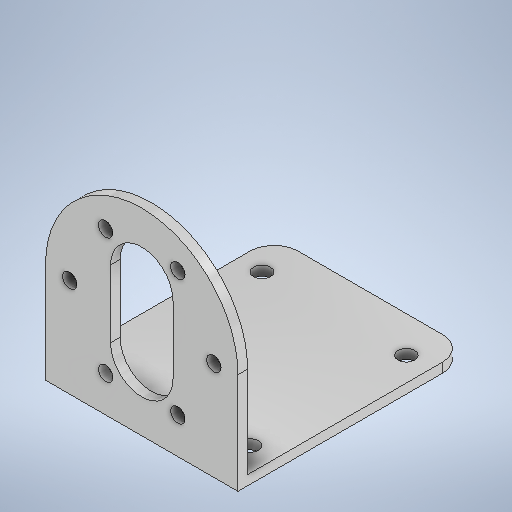
# Autodesk Inventor part: 520 DC Gear Motor Bracket
Saved by Autodesk Inventor 2025.2 (Build 292293000, 293)
## iProperties
Created: 2025-01-16
Part Number: 520 DC Gear Motor Bracket
Material: Generic
Document SubType Name: Modeling
Designer: Matt Tidd
Density: 1 g/cm^3
Appearance: Default
Author: Matt Tidd
Autodesk Inventor part; units mm, degrees
ref_plane "YZ Plane" through (0, 0, 0) normal (1, 0, 0) x (0, 1, 0)
ref_plane "XZ Plane" through (0, 0, 0) normal (0, 1, 0) x (-1, 0, 0)
ref_plane "XY Plane" through (0, 0, 0) normal (0, 0, 1) x (1, 0, 0)
sketch "Sketch1" plane through (0, 0, 0) normal (1, 0, 0) x (0, 1, 0)
  line L0 (0, 0) -> (2, 0)
  line L1 (2, 0) -> (2, -47.5)
  line L2 (2, -47.5) -> (0, -47.5)
  line L3 (0, -47.5) -> (0, 0)
  line L4 (0, 0) -> (41, 0)
  line L5 (41, 0) -> (41, -2)
  line L6 (41, -2) -> (0, -2)
  line L7 (0, -2) -> (0, 0)
  point P0 (2, -2)
  dimension "d0" = 2
  dimension "d1" = 47.5
  dimension "d2" = 41
  dimension "d3" = 2
  constraints: 16 end point, 4 parallel, 2 horizontal, 2 perpendicular
  measures "d0" distance of L1.end L2.end
  measures "d1" distance of L0.end L1.end
  measures "d2" distance of L5.end L6.end
  measures "d3" distance of L4.end L5.end
extrude "Extrusion1" add sketch "Sketch1" along normal blind 40
sketch "Sketch2" plane through (0, 0, 0) normal (0, 0, 1) x (1, 0, 0)
  line L0 (20, 27.5) -> (20, 13.5) construction
  line L1 (13.5, 27.5) -> (13.5, 13.5)
  line L2 (26.5, 13.5) -> (26.5, 27.5)
  arc A0 (26.5, 27.5) -> (13.5, 27.5) centre (20, 27.5) ccw
  arc A1 (13.5, 13.5) -> (26.5, 13.5) centre (20, 13.5) ccw
  circle A2 centre (35, 20.5) radius 1.5
  circle A3 centre (27.5, 33.4904) radius 1.5
  circle A4 centre (12.5, 33.4904) radius 1.5
  circle A5 centre (5, 20.5) radius 1.5
  circle A6 centre (12.5, 7.5096) radius 1.5
  circle A7 centre (27.5, 7.5096) radius 1.5
  point P0 (0, 0)
  point P1 (20, 20.5)
  point P2 (20, 20.5)
  dimension "d6" = 14
  dimension "d7" = 13
  dimension "d8" = 3
  dimension "d11" = 360
  constraints: 8 centre point, 8 end point, 4 point on circle, 4 tangent, 1 midpoint, 1 parallel, 1 vertical, 13 other
  measures "d6" distance of L0.start L0.end
  measures "d7" diameter of A1
  measures "d8" diameter of A2
extrude "Extrusion2" cut sketch "Sketch2" against normal blind 40
fillet "Fillet1" radius 20 2 edges at (40, 41, -1) (0, 41, -1)
sketch "Sketch3" plane through (0, 0, -47.5) normal (0, -1, 0) x (1, 0, 0)
  circle A0 centre (5, 40) radius 1.75
  line L0 (5, 40) -> (5, 7.5) construction
  line L1 (5, 40) -> (37.5, 40) construction
  line L2 (5, 7.5) -> (35, 7.5) construction
  circle A1 centre (5, 7.5) radius 1.75
  circle A2 centre (35, 40) radius 1.75
  circle A3 centre (35, 7.5) radius 1.75
  point P0 (0, 47.5)
  dimension "d16" = 3.5
  dimension "d17" = 32.5
  dimension "d18" = 90
  dimension "d19" = 30
  dimension "d20" = 90
  dimension "d23" = 32.5
  dimension "d26" = 30
  constraints: 6 end point, 4 centre point, 2 horizontal, 2 perpendicular, 2 vertical, 6 other
  measures "d16" diameter of A0
  measures "d17" distance of L0.start L0.end
  measures "d18" angle of L0 L1
  measures "d19" distance of L0.end L2.end
  measures "d20" angle of L2 L0
  measures "d23" distance of L0.start A1.centre
  measures "d26" distance of L0.start A2.centre
extrude "Extrusion3" cut sketch "Sketch3" against normal blind 40
fillet "Fillet2" radius 5 2 edges at (40, 1, -47.5) (0, 1, -47.5)
body "Solid1"
